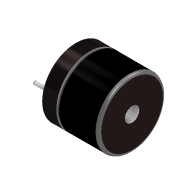
# Autodesk Inventor part: buzzer
Saved by Autodesk Inventor 2021 (Build 250183000, 183)
## iProperties
Created: 2021-06-23
Part Number: buzzer
Material: Generic
Document SubType Name: Modeling
Designer: Shrinidhi Patil
Density: 1 g/cm^3
Appearance: Aluminum - Polished
Author: Shrinidhi Patil
Autodesk Inventor part; units mm, degrees
ref_plane "YZ Plane" through (0, 0, 0) normal (1, 0, 0) x (0, 1, 0)
ref_plane "XZ Plane" through (0, 0, 0) normal (0, 1, 0) x (-1, 0, 0)
ref_plane "XY Plane" through (0, 0, 0) normal (0, 0, 1) x (1, 0, 0)
sketch "Sketch1" plane through (0, 0, 0) normal (0, 0, 1) x (1, 0, 0)
  point P0 (0, 0)
sketch "Sketch2" plane through (0, 0, 0) normal (0, 0, 1) x (1, 0, 0)
  line L0 (0, 0) -> (7, 0)
  line L1 (7, 0) -> (7, 6)
  line L2 (7, 6) -> (0, 6)
  line L3 (0, 6) -> (0, 0)
  line L4 (0, 0) -> (-0.5, 0)
  line L5 (-0.5, 0) -> (-0.5, 5.5)
  line L6 (-0.5, 5.5) -> (0, 5.5)
  line L7 (0, 5.5) -> (0, 0)
  line L8 (-0.5, 0) -> (-3, 0)
  line L9 (-3, 0) -> (-3, 6)
  line L10 (-3, 6) -> (-0.5, 6)
  line L11 (-0.5, 6) -> (-0.5, 0)
  constraints: 24 end point, 6 parallel, 3 horizontal, 3 perpendicular
revolve "Revolution1" add sketch "Sketch2" angle 360 about axis through (0, 0, 0) along (1, 0, 0)
sketch "Sketch3" plane through (-3, 0, 0) normal (-1, 0, 0) x (0, 0, 1)
  circle A0 centre (0, 0) radius 5.75
  dimension "d6" = 11.5
  constraints: 1 centre point, 1 coincident
  measures "d6" diameter of A0
extrude "Extrusion1" cut sketch "Sketch3" against normal blind 0.5
sketch "Sketch4" plane through (-2.5, 0, 0) normal (-1, 0, 0) x (0, 0, 1)
  line L0 (0, 0) -> (3.8, 0)
  circle A0 centre (3.8, 0) radius 0.3
  dimension "d9" = 3.8
  dimension "d10" = 0.6
  constraints: 2 end point, 1 centre point, 1 coincident, 1 horizontal
  measures "d9" distance of L0.start L0.end
  measures "d10" diameter of A0
extrude "Extrusion2" add sketch "Sketch4" along normal blind 4
sketch "Sketch5" plane through (-2.5, 0, 0) normal (-1, 0, 0) x (0, 0, 1)
  line L0 (0, 0) -> (-3.8, 0)
  circle A0 centre (-3.8, 0) radius 0.3
  dimension "d13" = 3.8
  dimension "d14" = 0.6
  constraints: 2 end point, 1 centre point, 1 coincident, 1 horizontal
  measures "d13" distance of L0.start L0.end
  measures "d14" diameter of A0
extrude "Extrusion3" add sketch "Sketch5" along normal blind 5.5
sketch "Sketch6" plane through (7, 0, 0) normal (1, 0, 0) x (0, 0, -1)
  circle A0 centre (0, 0) radius 1.3
  dimension "d17" = 2.6
  constraints: 1 centre point, 1 coincident
  measures "d17" diameter of A0
extrude "Extrusion4" cut sketch "Sketch6" against normal blind 2
fillet "Fillet1" radius 0.5 1 edges at (7, -6, 0)
body "Solid1"
